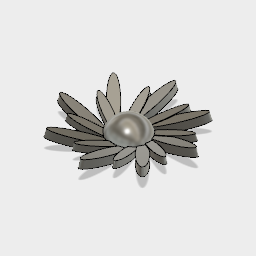
花 v1 (Autodesk Fusion 360 design; units mm, degrees)
Autodesk Fusion 360 part; units mm, degrees
sketch "草图1" plane through (0, 0, 0) normal (0, 1, 0) x (1, 0, 0)
  ellipse E0 centre (15, 0) end of major axis (25, 0) minor radius 2
  line L0 (5, 0) -> (25, 0)
  line L1 (15, -2) -> (15, 2)
extrude "拉伸1" add sketch "草图1" along normal blind 3 makes body 1
move_body "移动1" bodies 1 to x (0.965926, 0.258819, 0) y (-0.258819, 0.965926, 0) z (0, 0, 1) at (0.1704, -1.2941, 0)
box "长方体基本要素1" add length 7 width 6 height 6 placed x (0, 0, 1) y (1, 0, 0) z (0, 1, 0) at (-5, 0, -3) separate body makes body 2
pattern_circular "C-阵列1" count 8 over 360 about axis through (1, 6, 4) along (0, -1, 0) of bodies 1 makes body 3 at (14.7662, 3.2332, 12.9552) makes body 4 at (4.4019, 3.2332, 20.0664) makes body 5 at (-7.4062, 6.131, 17.2171) makes body 6 at (-15.0664, 3.2332, 7.4019) makes body 7 at (-12.7662, 3.2332, -4.9552) makes body 8 at (-2.4019, 6.131, -11.29) makes body 9 at (9.4062, 6.131, -9.2171)
copy_body "复制和粘贴实体1" bodies 1 3 4 5 6 7 8 9 makes body 10 makes body 11 makes body 12 makes body 13 makes body 14 makes body 15 makes body 16 makes body 17
scale "缩放1" factor 0.8 about (4.2235, 2.8978, 0) bodies 10 11 12 13 14 15 16 17
move_body "移动2" bodies 10 11 12 13 14 15 16 17 2 to x (0.906308, 0, 0.422618) y (0, 1, 0) z (-0.422618, 0, 0.906308) at (1.7842, 0, -0.0478)
sphere "球体基本要素1" add diameter 15 placed x (1, 0, 0) y (0, 1, 0) z (0, 0, 1) at (51, 69, 0) separate body makes body 18
move_body "MoveFace1" bodies 18 to x (1, 0, 0) y (0, 1, 0) z (0, 0, 1) at (-50.0865, -67.2775, 3.7056) on bodies 18
combine "合并1" operation add target body 18 tool bodies 15 8 16 9 17 1 10 3 11 4 12 5 13 6 14 7
box "长方体基本要素2" add length 40 width 35 height 17 placed x (0, 0, -1) y (-1, 0, 0) z (0, 1, 0) at (65, 0, 10) separate body makes body 19
move_body "移动3" bodies 18 to x (1, 0, 0) y (0, 1, 0) z (0, 0, 1) at (47.6181, 15.6167, -12.812)
combine "合并2" operation cut target body 18 tool bodies 19
hidden bodies 2
